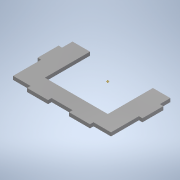
# Autodesk Inventor part: Plaat achter
Saved by Autodesk Inventor 2021 (Build 250183000, 183)
## iProperties
Manager: PJ / DCS
Company: Emmaüs Bovenbouw Aalter
Created: 2021-01-09
Part Number: Plaat achter
Material: S235
Catalog Web Link: http://emmausbovenbouw.op-weg.be/
Vendor: Emmaüsinstituut Bovenbouw Aalter
Document SubType Name: Modeling
Designer: Antho
Engineer: Declercq St.
Manufacturer: Standard
Standards Organization: Custom
Density: 7.86 g/cm^3
Appearance: Steel
Title: Algemene titel
Subject: Specifieke titel
Author: Antho
Keywords: Ruwe Ø xxxxx
Comments: Opmerking
Autodesk Inventor part; units mm, degrees
ref_plane "YZ Plane" through (0, 0, 0) normal (1, 0, 0) x (0, 1, 0)
ref_plane "XZ Plane" through (0, 0, 0) normal (0, 1, 0) x (-1, 0, 0)
ref_plane "XY Plane" through (0, 0, 0) normal (0, 0, 1) x (1, 0, 0)
sketch "Sketch1" plane through (0, 0, 0) normal (0, 0, 1) x (1, 0, 0)
  line L0 (0, 2.8582) -> (0, -2.8582) construction
  line L1 (-5.7775, 0) -> (5.7775, 0) construction
  line L2 (-75, -70.5) -> (75, -70.5)
  line L3 (75, -70.5) -> (75, 70.5)
  line L4 (75, 70.5) -> (-75, 70.5)
  line L5 (-75, 70.5) -> (-75, -70.5)
  line L6 (-75, -70.5) -> (75, 70.5) construction
  line L7 (75, -70.5) -> (-75, 70.5) construction
  point P0 (0, 0)
  point P1 (0, 0)
  dimension "d0" = 150
  dimension "d1" = 141
  constraints: 16 end point, 4 midpoint, 2 horizontal, 2 parallel, 1 coincident, 1 perpendicular, 1 vertical
  measures "d0" distance of L4.end L3.end
  measures "d1" distance of L3.end L2.end
extrude "Extrusion1" add sketch "Sketch1" along normal blind 5
sketch "Sketch2" plane through (0, 0, 5) normal (0, 0, 1) x (1, 0, 0)
  line L0 (-75, -70.5) -> (75, -70.5) projected
  line L1 (0, -70.5) -> (-15, -70.5)
  line L2 (-15, -70.5) -> (15, -70.5)
  line L3 (15, -70.5) -> (45, -70.5)
  line L4 (-15, -70.5) -> (-45, -70.5)
  line L5 (-15, -70.5) -> (15, -70.5)
  line L6 (15, -70.5) -> (15, -65.5)
  line L7 (15, -65.5) -> (-15, -65.5)
  line L8 (-15, -65.5) -> (-15, -70.5)
  line L9 (75, -70.5) -> (75, 70.5) projected
  line L10 (45, -70.5) -> (75, -70.5)
  line L11 (75, -70.5) -> (75, -65.5)
  line L12 (75, -65.5) -> (45, -65.5)
  line L13 (45, -65.5) -> (45, -70.5)
  line L14 (-75, 70.5) -> (-75, -70.5) projected
  line L15 (-45, -70.5) -> (-75, -70.5)
  line L16 (-75, -70.5) -> (-75, -65.5)
  line L17 (-75, -65.5) -> (-45, -65.5)
  line L18 (-45, -65.5) -> (-45, -70.5)
  line L19 (75, -70.5) -> (75, -55.5)
  line L20 (75, -55.5) -> (75, -25.5)
  line L21 (75, -25.5) -> (75, 4.5)
  line L22 (75, 4.5) -> (75, 34.5)
  line L23 (75, 34.5) -> (75, 64.5)
  line L24 (75, -25.5) -> (70, -25.5)
  line L25 (70, -25.5) -> (70, 4.5)
  line L26 (70, 4.5) -> (75, 4.5)
  line L27 (75, 4.5) -> (75, -25.5)
  line L28 (75, 70.5) -> (-75, 70.5) projected
  line L29 (75, 34.5) -> (70, 34.5)
  line L30 (70, 34.5) -> (70, 70.5)
  line L31 (70, 70.5) -> (75, 70.5)
  line L32 (75, 70.5) -> (75, 34.5)
  line L33 (-75, -25.5) -> (-70, -25.5)
  line L34 (-70, -25.5) -> (-70, 4.5)
  line L35 (-70, 4.5) -> (-75, 4.5)
  line L36 (-75, 4.5) -> (-75, -25.5)
  line L37 (-75, 34.5) -> (-70, 34.5)
  line L38 (-70, 34.5) -> (-70, 70.5)
  line L39 (-70, 70.5) -> (-75, 70.5)
  line L40 (-75, 70.5) -> (-75, 34.5)
  line L41 (0, 70.5) -> (-15, 70.5)
  line L42 (-15, 70.5) -> (15, 70.5)
  line L43 (15, 70.5) -> (45, 70.5)
  line L44 (-15, 70.5) -> (-45, 70.5)
  line L45 (-75, 70.5) -> (-45, 70.5)
  line L46 (-45, 70.5) -> (-45, 65.5)
  line L47 (-45, 65.5) -> (-75, 65.5)
  line L48 (-75, 65.5) -> (-75, 70.5)
  line L49 (-15, 70.5) -> (15, 70.5)
  line L50 (15, 70.5) -> (15, 65.5)
  line L51 (15, 65.5) -> (-15, 65.5)
  line L52 (-15, 65.5) -> (-15, 70.5)
  line L53 (45, 70.5) -> (75, 70.5)
  line L54 (75, 70.5) -> (75, 65.5)
  line L55 (75, 65.5) -> (45, 65.5)
  line L56 (45, 65.5) -> (45, 70.5)
  line L57 (-75, -25.5) -> (-70, -25.5)
  line L58 (-70, -25.5) -> (-70, -70.5)
  line L59 (-70, -70.5) -> (-75, -70.5)
  line L60 (-75, -70.5) -> (-75, -25.5)
  line L61 (-75, 4.5) -> (-70, 4.5)
  line L62 (-70, 4.5) -> (-70, 34.5)
  line L63 (-70, 34.5) -> (-75, 34.5)
  line L64 (-75, 34.5) -> (-75, 4.5)
  line L65 (70, 34.5) -> (75, 34.5)
  line L66 (75, 34.5) -> (75, 4.5)
  line L67 (75, 4.5) -> (70, 4.5)
  line L68 (70, 4.5) -> (70, 34.5)
  line L69 (70, -25.5) -> (75, -25.5)
  line L70 (75, -25.5) -> (75, -70.5)
  line L71 (75, -70.5) -> (70, -70.5)
  line L72 (70, -70.5) -> (70, -25.5)
  point P0 (0, 0)
  point P1 (75, 4.5)
  point P2 (-70, 70.5)
  point P3 (-75, 4.5)
  point P4 (70, 65.5)
  point P5 (-70, 65.5)
  point P6 (-70, -65.5)
  point P7 (70, -65.5)
  dimension "d4" = 15
  dimension "d5" = 30
  dimension "d6" = 30
  dimension "d7" = 30
  dimension "d8" = 30
  dimension "d9" = 5
  dimension "d10" = 15
  dimension "d11" = 30
  dimension "d14" = 30
  dimension "d15" = 5
  dimension "d16" = 5
  dimension "d17" = 5
  dimension "d24" = 15
  dimension "d25" = 30
  dimension "d26" = 30
  dimension "d27" = 30
  dimension "d28" = 5
  dimension "d32" = 5
  dimension "d33" = 30
  dimension "d34" = 30
  constraints: 138 end point, 29 point on line, 28 parallel, 14 horizontal, 14 perpendicular, 2 midpoint
  measures "d4" distance of L1.start L1.end
  measures "d5" distance of L1.end L2.end
  measures "d6" distance of L2.end L3.end
  measures "d7" distance of L1.end L4.end
  measures "d8" distance of L7.end L6.end
  measures "d9" distance of L6.end L5.end
  measures "d10" distance of L10.end L19.end
  measures "d11" distance of L19.end L20.end
  measures "d14" distance of L22.end L23.end
  measures "d15" distance of L25.end L26.end
  measures "d16" distance of L30.end L31.end
  measures "d17" distance of L35.end L34.end
  measures "d24" distance of L41.start L41.end
  measures "d25" distance of L41.end L42.end
  measures "d26" distance of L42.end L43.end
  measures "d27" distance of L41.end L44.end
  measures "d28" distance of L45.end L46.end
  measures "d32" distance between parallel lines of L60 L58
  measures "d33" distance between parallel lines of L24 L26
  measures "d34" distance between parallel lines of L29 L26
extrude "Extrusion2" cut sketch "Sketch2" against normal blind 8 contours L14 L17 L58 L0 | L58 L17 L18 L0 | L14 L33 L58 L17 | L8 L7 L6 L0 | L14 L37 L62 L35 | L14 L28 L38 L47 | L13 L12 L72 L0 | L38 L28 L46 L47 | L72 L12 L9 L0 | L72 L24 L9 L12 | L28 L50 L51 L52 | L68 L29 L9 L26 | L55 L56 L28 L30 | L30 L28 L9 L55
sketch "Sketch3" plane through (0, 0, 5) normal (0, 0, 1) x (1, 0, 0)
  line L0 (-45, -45) -> (45, -45)
  line L1 (45, -45) -> (45, 45)
  line L2 (45, 45) -> (-45, 45)
  line L3 (-45, 45) -> (-45, -45)
  line L4 (-45, -45) -> (45, 45) construction
  line L5 (45, -45) -> (-45, 45) construction
  point P0 (0, 0)
  dimension "d20" = 90
  dimension "d21" = 90
  constraints: 12 end point, 2 midpoint, 2 parallel, 1 horizontal, 1 perpendicular
  measures "d20" distance of L2.end L1.end
  measures "d21" distance of L1.end L0.end
extrude "Extrusion3" cut sketch "Sketch3" against normal blind 8
sketch "Sketch4" plane through (0, 0, 5) normal (0, 0, 1) x (1, 0, 0)
  line L0 (75, 34.5) -> (75, 65.5) projected
  line L1 (75, 65.5) -> (75, 21.5)
  line L2 (75, 21.5) -> (-125.9097, 21.5)
  line L3 (-125.9097, 21.5) -> (-125.9097, 76.2896)
  line L4 (-125.9097, 76.2896) -> (75, 76.2896)
  line L5 (75, 76.2896) -> (75, 21.5)
  point P0 (0, 0)
  dimension "d29" = 44
  constraints: 10 end point, 2 parallel, 1 collinear, 1 horizontal, 1 perpendicular
  measures "d29" distance of L0.end L1.end
extrude "Extrusion4" cut sketch "Sketch4" against normal blind 15
sketch "Sketch5" plane through (45, 21.5, 5) normal (0, 1, 0) x (1, 0, 0)
  line L0 (36.0509, -17.7295) -> (-126.227, -17.7295)
  line L1 (-126.227, -17.7295) -> (-126.227, 31.9582)
  line L2 (-126.227, 31.9582) -> (36.0509, 31.9582)
  line L3 (36.0509, 31.9582) -> (36.0509, -17.7295)
  point P0 (-45, 5)
  constraints: 8 end point, 2 parallel, 1 horizontal, 1 perpendicular
extrude "Extrusion5" cut sketch "Sketch5" against normal blind 2
body "Solid1"
